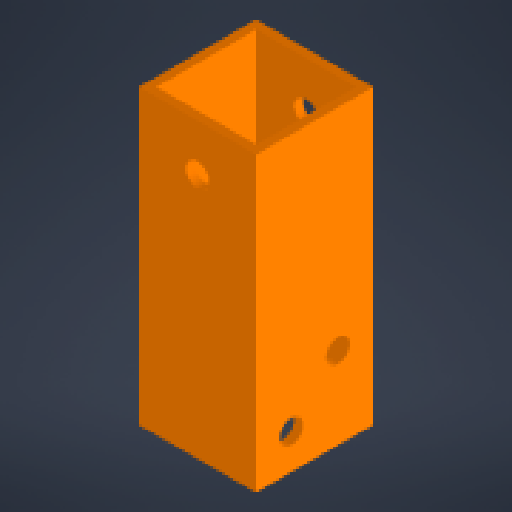
# Autodesk Inventor part: square_box_side_section
Saved by Autodesk Inventor 2024 (Build 280153000, 153)
## iProperties
Created: 2023-04-16
Part Number: square_box_side_section
Material: Типовые
Document SubType Name: Modeling
Designer: user
Density: 1 g/cm^3
Appearance: По умолчанию
Author: user
Autodesk Inventor part; units mm, degrees
ref_plane "YZ Plane" through (0, 0, 0) normal (1, 0, 0) x (0, 1, 0)
ref_plane "XZ Plane" through (0, 0, 0) normal (0, 1, 0) x (-1, 0, 0)
ref_plane "XY Plane" through (0, 0, 0) normal (0, 0, 1) x (1, 0, 0)
sketch "Эскиз1" plane through (0, 0, 0) normal (0, 0, 1) x (1, 0, 0)
  line L0 (-20, 0) -> (0, 0) construction
  line L1 (0, -380) -> (0, 0) construction
  line L2 (0, 0) -> (-20, 0)
  line L3 (-20, 0) -> (-20, -20)
  line L4 (-20, -20) -> (0, -20)
  line L5 (0, -20) -> (0, 0)
  line L6 (-18.5, -1.5) -> (-1.5, -1.5)
  line L7 (-1.5, -1.5) -> (-1.5, -18.5)
  line L8 (-1.5, -18.5) -> (-18.5, -18.5)
  line L9 (-18.5, -18.5) -> (-18.5, -1.5)
  point P0 (-10, -18.5)
  point P1 (-10, -20)
  point P2 (-1.5, -10)
  point P3 (0, -10)
  dimension "d0" = 1.5
  constraints: 16 end point, 5 perpendicular, 4 midpoint, 4 parallel, 2 horizontal, 1 horizontal alignment, 1 vertical alignment
  measures "d0" horizontal distance of L4.end L7.end
extrude "Выдавливание1" add sketch "Эскиз1" along normal blind 50
sketch "Эскиз2" plane through (0, -20, 0) normal (1, 0, 0) x (0, 0, -1)
  circle A0 centre (-6, 6) radius 2
  circle A1 centre (-14, 14) radius 2
  circle A2 centre (14, 14) radius 2 construction
  circle A3 centre (6, 6) radius 2 construction
  line L0 (0, -360) -> (0, 20) construction
  line L1 (6, 6) -> (0, 6) construction
  line L2 (14, 14) -> (0, 14) construction
  line L3 (0, 14) -> (-14, 14) construction
  line L4 (-6, 6) -> (0, 6) construction
  constraints: 8 end point, 3 collinear, 3 perpendicular, 2 centre point, 2 equal radius, 2 horizontal alignment, 2 point on line
extrude "Выдавливание2" cut sketch "Эскиз2" against normal through all
sketch "Эскиз3" plane through (-20, 0, 0) normal (0, 1, 0) x (1, 0, 0)
  circle A0 centre (10, -42) radius 2
  line L0 (20, -50) -> (0, -50) projected
  point P0 (20, 0)
  point P1 (10, -50)
  dimension "d5" = 8
  dimension "d8" = 4
  constraints: 1 centre point, 1 midpoint, 1 vertical alignment
  measures "d5" vertical distance of L0.start A0.centre
  measures "d8" diameter of A0
extrude "Выдавливание3" cut sketch "Эскиз3" against normal through all
